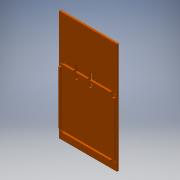
# Autodesk Inventor part: chassis-akksi
Saved by Autodesk Inventor 2019 (Build 230136000, 136)
## iProperties
Created: 2019-02-14
Part Number: chassis-akksi
Material: Generic
Document SubType Name: Modeling
Designer: izsoandras
Density: 1 g/cm^3
Appearance: Default
Author: izsoandras
Autodesk Inventor part; units mm, degrees
ref_plane "YZ Plane" through (0, 0, 0) normal (1, 0, 0) x (0, 1, 0)
ref_plane "XZ Plane" through (0, 0, 0) normal (0, 1, 0) x (-1, 0, 0)
ref_plane "XY Plane" through (0, 0, 0) normal (0, 0, 1) x (1, 0, 0)
sketch "Sketch1" plane through (0, 0, 0) normal (0, 0, 1) x (1, 0, 0)
  line L0 (59, 131.5) -> (-36.0094, 131.5)
  line L1 (-36.0094, 131.5) -> (-36.0094, -49.2144)
  line L2 (-36.0094, -49.2144) -> (59, -49.2144)
  line L3 (59, -49.2144) -> (59, 131.5)
  point P0 (0, 0)
  point P1 (-36, 131.5)
  point P2 (59.0094, -49.2144)
  constraints: 8 end point, 2 parallel, 1 horizontal, 1 perpendicular, 4 other
extrude "Extrusion1" add sketch "Sketch1" along normal blind 3
sketch "Sketch2" plane through (0, 0, 3) normal (0, 0, 1) x (1, 0, 0)
  line L0 (16.62, 69.08) -> (14.03, 69.08)
  line L1 (14.03, 69.08) -> (14.03, 48.08)
  line L2 (14.03, 48.08) -> (16.62, 48.08)
  line L3 (16.62, 48.08) -> (16.62, 69.08)
  line L4 (-6.41, 48.08) -> (-6.41, 69.08)
  line L5 (-6.41, 69.08) -> (-9, 69.08)
  line L6 (-9, 69.08) -> (-9, 48.08)
  line L7 (-9, 48.08) -> (-6.41, 48.08)
  line L8 (59, 131.5) -> (-36.0094, 131.5)
  line L9 (-36.0094, 131.5) -> (-36.0094, -49.2144)
  line L10 (-36.0094, -49.2144) -> (59, -49.2144)
  line L11 (59, -49.2144) -> (59, 131.5)
  line L12 (17.12, 69.58) -> (13.53, 69.58)
  line L13 (13.53, 69.58) -> (13.53, 47.58)
  line L14 (13.53, 47.58) -> (17.12, 47.58)
  line L15 (17.12, 47.58) -> (17.12, 69.58)
  line L16 (-5.91, 69.58) -> (-9.5, 69.58)
  line L17 (-9.5, 69.58) -> (-9.5, 47.58)
  line L18 (-9.5, 47.58) -> (-5.91, 47.58)
  line L19 (-5.91, 47.58) -> (-5.91, 69.58)
  circle A0 centre (55.5094, 59.3944) radius 1.5
  circle A1 centre (55.5094, -36.7144) radius 1.5
  circle A2 centre (-32.5094, -36.7144) radius 1.5
  circle A3 centre (-32.5094, 59.3944) radius 1.5
  point P0 (0, 0)
extrude "Extrusion2" cut sketch "Sketch2" against normal up to next contours L3 L2 L1 L0 | L7 L6 L5 L4 | L15 L14 L13 L12 | L19 L18 L17 L16 | A0 | A1 | A2 | A3
sketch "Sketch3" plane through (0, 0, 3) normal (0, 0, 1) x (1, 0, 0)
  line L0 (-34.195, 54.8944) -> (-31.195, 54.8944) projected
  line L1 (-31.195, 54.8944) -> (-31.195, -32.2144) projected
  line L2 (-31.195, -32.2144) -> (-34.195, -32.2144) projected
  line L3 (-34.195, -32.2144) -> (-34.195, 54.8944) projected
  line L4 (54.195, 54.8944) -> (57.195, 54.8944) projected
  line L5 (57.195, 54.8944) -> (57.195, -32.2144) projected
  line L6 (57.195, -32.2144) -> (54.195, -32.2144) projected
  line L7 (54.195, -32.2144) -> (54.195, 54.8944) projected
  line L8 (-28.0094, -35.4) -> (51.0094, -35.4) projected
  line L9 (51.0094, -35.4) -> (51.0094, -38.4) projected
  line L10 (51.0094, -38.4) -> (-28.0094, -38.4) projected
  line L11 (-28.0094, -38.4) -> (-28.0094, -35.4) projected
  line L12 (51.0094, 61.08) -> (51.0094, 58.08) projected
  line L13 (-28.0094, 58.08) -> (-28.0094, 61.08) projected
  line L14 (17.12, 47.58) -> (17.12, 69.58) projected
  line L15 (51.0094, 58.08) -> (17.12, 58.08)
  line L16 (17.12, 58.08) -> (17.12, 61.08)
  line L17 (17.12, 61.08) -> (51.0094, 61.08)
  line L18 (51.0094, 61.08) -> (51.0094, 58.08)
  line L19 (13.53, 47.58) -> (13.53, 69.58) projected
  line L20 (-5.91, 69.58) -> (-5.91, 47.58) projected
  line L21 (13.53, 58.08) -> (-5.91, 58.08)
  line L22 (-5.91, 58.08) -> (-5.91, 61.08)
  line L23 (-5.91, 61.08) -> (13.53, 61.08)
  line L24 (13.53, 61.08) -> (13.53, 58.08)
  line L25 (-9.5, 47.58) -> (-9.5, 69.58) projected
  line L26 (-28.0094, 58.08) -> (-9.5, 58.08)
  line L27 (-9.5, 58.08) -> (-9.5, 61.08)
  line L28 (-9.5, 61.08) -> (-28.0094, 61.08)
  line L29 (-28.0094, 61.08) -> (-28.0094, 58.08)
  point P0 (0, 0)
  constraints: 24 end point, 7 point on line, 6 parallel, 3 horizontal, 3 perpendicular
extrude "Extrusion3" add sketch "Sketch3" along normal blind 3
sketch "Sketch4" plane through (0, 0, 0) normal (0, 0, -1) x (-1, 0, 0)
  line L0 (16, 116.5) -> (36, 116.5) projected
  line L1 (36, 116.5) -> (36, -41.136) projected
  line L2 (36, -41.136) -> (16, -41.136) projected
  line L3 (16, -41.136) -> (16, 116.5) projected
  line L4 (-59, 116.5) -> (-39, 116.5) projected
  line L5 (-39, 116.5) -> (-39, -41.136) projected
  line L6 (-39, -41.136) -> (-59, -41.136) projected
  line L7 (-59, -41.136) -> (-59, 116.5) projected
  line L8 (14.5, -41.136) -> (17.5, -41.136)
  line L9 (17.5, -41.136) -> (17.5, 116.5)
  line L10 (17.5, 116.5) -> (14.5, 116.5)
  line L11 (14.5, 116.5) -> (14.5, -41.136)
  line L12 (-37.5, 116.5) -> (-40.5, 116.5)
  line L13 (-40.5, 116.5) -> (-40.5, -41.136)
  line L14 (-40.5, -41.136) -> (-37.5, -41.136)
  line L15 (-37.5, -41.136) -> (-37.5, 116.5)
  point P0 (0, 0)
  dimension "d13" = 1.5
  dimension "d14" = 1.5
  dimension "d15" = 1.5
  dimension "d16" = 1.5
  constraints: 16 end point, 4 parallel, 3 point on line, 2 horizontal, 2 perpendicular
  measures "d13" distance between parallel lines of L3 L11
  measures "d14" distance between parallel lines of L3 L9
  measures "d15" distance between parallel lines of L5 L15
  measures "d16" distance between parallel lines of L5 L13
extrude "Extrusion4" add sketch "Sketch4" along normal blind 6.7 contours L0 L9 L2 L3 | L3 L8 L11 L10 | L4 L5 L6 L13 | L12 L15 L14 L5
sketch "Sketch5" plane through (0, 0, 0) normal (0, 0, -1) x (-1, 0, 0)
  line L0 (-37, -32) -> (-37, 31) projected
  line L1 (9, 32) -> (9, -32) projected
  line L2 (14.5, 116.5) -> (14.5, -41.136) projected
  line L3 (-37, 24.2384) -> (14.5, 24.2384)
  line L4 (14.5, 24.2384) -> (14.5, 21.2384)
  line L5 (14.5, 21.2384) -> (-37, 21.2384)
  line L6 (-37, 21.2384) -> (-37, 24.2384)
  line L7 (-37.5, 116.5) -> (-37.5, -41.136) projected
  line L8 (14.5, -16.674) -> (-37.5, -16.674)
  line L9 (-37.5, -16.674) -> (-37.5, -19.674)
  line L10 (-37.5, -19.674) -> (14.5, -19.674)
  line L11 (14.5, -19.674) -> (14.5, -16.674)
  point P0 (0, 0)
  dimension "d20" = 3
  dimension "d21" = 3
  constraints: 16 end point, 4 parallel, 4 point on line, 2 horizontal, 2 perpendicular
  measures "d20" distance between parallel lines of L10 L8
  measures "d21" distance between parallel lines of L3 L5
extrude "Extrusion5" add sketch "Sketch5" along normal blind 1.7 contours L0 L3 L1 L5 | L8 L1 L10 L0 | L0 L10 L7 L8 | L1 L3 L2 L5 | L8 L2 L10 L1
equation "\"d14\" = d13"
equation "\"d15\" = d13"
equation "\"d16\" = d13"
body "Solid1"
